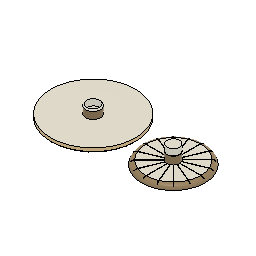
CAKE TABLE (Autodesk Fusion 360 design; units mm, degrees)
part number: 2026-07-16-17-54-16-538
Autodesk Fusion 360 part; units mm, degrees
sketch "Sketch1" plane through (0, 0, 0) normal (0, 1, 0) x (1, 0, 0)
  circle A0 centre (0, 0) radius 75
  dimension "d1" = 150
  constraint coincident A0.centre origin
  measures "d1" diameter of A0
extrude "Extrude1" add sketch "Sketch1" along normal blind 10 makes body 1
ref_plane "WorkPlane1" through (0, 10, 0) normal (0, 1, 0) x (1, 0, 0)
sketch "Sketch2" plane through (0, 10, 0) normal (0, 1, 0) x (1, 0, 0)
  line L0 (0, 0) -> (1, 0)
  line L1 (1, 0) -> (1, -74.9885)
  line L2 (1, -74.9885) -> (0, -74.9885)
  line L3 (0, -74.9885) -> (0, 0)
  line L4 (28.6969, -69.2803) -> (0, 0)
  line L5 (0, 0) -> (0.9239, 0.3827)
  line L6 (29.6207, -68.8977) -> (28.6969, -69.2803)
  line L7 (0.9239, 0.3827) -> (29.6207, -68.8977)
  line L8 (53.0249, -53.0249) -> (0, 0)
  line L9 (0, 0) -> (0.7071, 0.7071)
  line L10 (53.732, -52.3178) -> (53.0249, -53.0249)
  line L11 (0.7071, 0.7071) -> (53.732, -52.3178)
  line L12 (69.2803, -28.6969) -> (0, 0)
  line L13 (0, 0) -> (0.3827, 0.9239)
  line L14 (69.663, -27.773) -> (69.2803, -28.6969)
  line L15 (0.3827, 0.9239) -> (69.663, -27.773)
  line L16 (74.9885, 0) -> (0, 0)
  line L17 (0, 0) -> (0, 1)
  line L18 (74.9885, 1) -> (74.9885, 0)
  line L19 (0, 1) -> (74.9885, 1)
  line L20 (69.2803, 28.6969) -> (0, 0)
  line L21 (0, 0) -> (-0.3827, 0.9239)
  line L22 (68.8977, 29.6207) -> (69.2803, 28.6969)
  line L23 (-0.3827, 0.9239) -> (68.8977, 29.6207)
  line L24 (53.0249, 53.0249) -> (0, 0)
  line L25 (0, 0) -> (-0.7071, 0.7071)
  line L26 (52.3178, 53.732) -> (53.0249, 53.0249)
  line L27 (-0.7071, 0.7071) -> (52.3178, 53.732)
  line L28 (28.6969, 69.2803) -> (0, 0)
  line L29 (0, 0) -> (-0.9239, 0.3827)
  line L30 (27.773, 69.663) -> (28.6969, 69.2803)
  line L31 (-0.9239, 0.3827) -> (27.773, 69.663)
  line L32 (0, 74.9885) -> (0, 0)
  line L33 (0, 0) -> (-1, 0)
  line L34 (-1, 74.9885) -> (0, 74.9885)
  line L35 (-1, 0) -> (-1, 74.9885)
  line L36 (-28.6969, 69.2803) -> (0, 0)
  line L37 (0, 0) -> (-0.9239, -0.3827)
  line L38 (-29.6207, 68.8977) -> (-28.6969, 69.2803)
  line L39 (-0.9239, -0.3827) -> (-29.6207, 68.8977)
  line L40 (-53.0249, 53.0249) -> (0, 0)
  line L41 (0, 0) -> (-0.7071, -0.7071)
  line L42 (-53.732, 52.3178) -> (-53.0249, 53.0249)
  line L43 (-0.7071, -0.7071) -> (-53.732, 52.3178)
  line L44 (-69.2803, 28.6969) -> (0, 0)
  line L45 (0, 0) -> (-0.3827, -0.9239)
  line L46 (-69.663, 27.773) -> (-69.2803, 28.6969)
  line L47 (-0.3827, -0.9239) -> (-69.663, 27.773)
  line L48 (-74.9885, 0) -> (0, 0)
  line L49 (0, 0) -> (0, -1)
  line L50 (-74.9885, -1) -> (-74.9885, 0)
  line L51 (0, -1) -> (-74.9885, -1)
  line L52 (-69.2803, -28.6969) -> (0, 0)
  line L53 (0, 0) -> (0.3827, -0.9239)
  line L54 (-68.8977, -29.6207) -> (-69.2803, -28.6969)
  line L55 (0.3827, -0.9239) -> (-68.8977, -29.6207)
  line L56 (-53.0249, -53.0249) -> (0, 0)
  line L57 (0, 0) -> (0.7071, -0.7071)
  line L58 (-52.3178, -53.732) -> (-53.0249, -53.0249)
  line L59 (0.7071, -0.7071) -> (-52.3178, -53.732)
  line L60 (-28.6969, -69.2803) -> (0, 0)
  line L61 (0, 0) -> (0.9239, -0.3827)
  line L62 (-27.773, -69.663) -> (-28.6969, -69.2803)
  line L63 (0.9239, -0.3827) -> (-27.773, -69.663)
  dimension "d5" = 1
  dimension "d7" = 360
  constraint horizontal L0
  constraint vertical L1
  constraint horizontal L2
  constraint vertical L3
  constraint coincident L0.start L3.end
  measures "d5" distance of L0.start L0.end
extrude "Extrude2" cut sketch "Sketch2" against normal blind 3 contours L1 L4 L6 L7 L8 | L7 L8 L10 L11 L12 | L11 L12 L14 L15 L16 | L3 L59 L60 L62 L63 | L55 L56 L58 L59 L60 | L51 L52 L54 L55 L56 | L1 L2 L3 L4 L63 | L15 L16 L18 L19 L20 | L19 L20 L22 L23 L24 | L23 L24 L26 L27 L28 | L27 L28 L30 L31 L32 | L31 L32 L34 L35 L36 | L35 L36 L38 L39 L40 | L39 L40 L42 L43 L44 | L43 L44 L46 L47 L48 | L47 L48 L50 L51 L52 bodies 1
sketch "Sketch3" plane through (0, 10, 0) normal (0, 1, 0) x (1, 0, 0)
  circle A0 centre (0, 0) radius 15
  dimension "d10" = 30
  constraint coincident A0.centre origin
  measures "d10" diameter of A0
extrude "Extrude3" add sketch "Sketch3" along normal blind 20 separate body makes body 2
fillet "Fillet1" radius 10.5 1 edges at (-69.9246, 10, 27.1212) on bodies 1
move_body "Move1" bodies 2 to x (1, 0, 0) y (0, 1, 0) z (0, 0, 1) at (0, -5, 0)
ref_plane "WorkPlane2" through (0, 30, 0) normal (0, 1, 0) x (1, 0, 0)
sketch "Sketch4" plane through (0, 30, 0) normal (0, 1, 0) x (1, 0, 0)
  circle A0 centre (0, 0) radius 17.5
  dimension "d18" = 35
  constraint coincident A0.centre origin
  measures "d18" diameter of A0
extrude "Extrude4" add sketch "Sketch4" along normal blind 20 separate body makes body 3
fillet "Fillet3" radius 3.5 1 edges at (-16.3157, 30, 6.3283) on bodies 3
move_body "Move2" bodies 3 to x (1, 0, 0) y (0, 1, 0) z (0, 0, 1) at (0, -2, 0)
extrude "Extrude5" add 1 faces at (3.8315, 25, -5.6199) along direction (0, 1, 0) blind 9 on bodies 2 bodies 2 3
ref_plane "WorkPlane3" through (0, 48, 0) normal (0, 1, 0) x (1, 0, 0)
sketch "Sketch5" plane through (0, 48, 0) normal (0, 1, 0) x (1, 0, 0)
  circle A0 centre (0, 0) radius 99.8908
  constraint coincident A0.centre origin
extrude "Extrude6" add sketch "Sketch5" along normal blind 10 separate body makes body 4
fillet "Fillet4" radius 2.5 1 edges at (-93.1309, 58, 36.1221) on bodies 4
ref_plane "WorkPlane4" through (0, 58, 0) normal (0, 1, 0) x (1, 0, 0)
sketch "Sketch6" plane through (0, 58, 0) normal (0, 1, 0) x (1, 0, 0)
  circle A0 centre (0, 0) radius 17.4885
  circle A1 centre (0, 0) radius 16.8218
  line L0 (0.5452, -17.48) -> (-1.5075, -17.48)
  line L1 (-1.5075, -17.48) -> (-1.5075, -98.7314)
  line L2 (-1.5075, -98.7314) -> (0.5452, -98.7314)
  line L3 (0.5452, -98.7314) -> (0.5452, -17.48)
  line L4 (63.881, -75.2822) -> (11.6536, -13.04)
  line L5 (11.6536, -13.04) -> (10.0812, -14.3595)
  line L6 (10.0812, -14.3595) -> (62.3085, -76.6017)
  line L7 (62.3085, -76.6017) -> (63.881, -75.2822)
  line L8 (97.3262, -16.6076) -> (17.3092, -2.4985)
  line L9 (17.3092, -2.4985) -> (16.9527, -4.52)
  line L10 (16.9527, -4.52) -> (96.9697, -18.6291)
  line L11 (96.9697, -18.6291) -> (97.3262, -16.6076)
  line L12 (85.2313, 49.8379) -> (14.8656, 9.2122)
  line L13 (14.8656, 9.2122) -> (15.8919, 7.4345)
  line L14 (15.8919, 7.4345) -> (86.2577, 48.0602)
  line L15 (86.2577, 48.0602) -> (85.2313, 49.8379)
  line L16 (33.2558, 92.9637) -> (5.4662, 16.6123)
  line L17 (5.4662, 16.6123) -> (7.3951, 15.9103)
  line L18 (7.3951, 15.9103) -> (35.1847, 92.2616)
  line L19 (35.1847, 92.2616) -> (33.2558, 92.9637)
  line L20 (-34.2805, 92.5907) -> (-6.4909, 16.2394)
  line L21 (-6.4909, 16.2394) -> (-4.562, 16.9415)
  line L22 (-4.562, 16.9415) -> (-32.3516, 93.2928)
  line L23 (-32.3516, 93.2928) -> (-34.2805, 92.5907)
  line L24 (-85.7765, 48.8935) -> (-15.4108, 8.2679)
  line L25 (-15.4108, 8.2679) -> (-14.3844, 10.0455)
  line L26 (-14.3844, 10.0455) -> (-84.7502, 50.6712)
  line L27 (-84.7502, 50.6712) -> (-85.7765, 48.8935)
  line L28 (-97.1368, -17.6815) -> (-17.1198, -3.5723)
  line L29 (-17.1198, -3.5723) -> (-17.4763, -1.5508)
  line L30 (-17.4763, -1.5508) -> (-97.4932, -15.6599)
  line L31 (-97.4932, -15.6599) -> (-97.1368, -17.6815)
  line L32 (-63.0457, -75.9831) -> (-10.8183, -13.7409)
  line L33 (-10.8183, -13.7409) -> (-12.3908, -12.4215)
  line L34 (-12.3908, -12.4215) -> (-64.6181, -74.6637)
  line L35 (-64.6181, -74.6637) -> (-63.0457, -75.9831)
  dimension "d33" = 360
  constraint coincident A0.centre A1.centre
  constraint concentric A0 A1
  constraint horizontal L0
  constraint vertical L1
  constraint horizontal L2
  constraint vertical L3
  constraint coincident A0 L0.start
extrude "Extrude7" cut sketch "Sketch6" against normal blind 1 contours A0 L8 L9 L10 L11 | A0 L12 L13 L14 L15 | A0 L4 L5 L6 L7 | A0 L16 L17 L18 L19 | A0 L0 L1 L2 L3 | A0 L20 L21 L22 L23 | A0 L32 L33 L34 L35 | A0 L24 L25 L26 L27 | A0 L28 L29 L30 L31 bodies 4
extrude "Extrude8" cut sketch "Sketch6" against normal blind 0.5 contours A0 L0 L5 L9 L13 L17 L21 L25 L29 L33 bodies 4
sketch "Sketch7" plane through (0, 58, 0) normal (0, 1, 0) x (1, 0, 0)
  circle A0 centre (0, 37.1794) radius 4.1177
  circle A1 centre (-23.8985, 28.4811) radius 4.1177
  circle A2 centre (-36.6146, 6.4561) radius 4.1177
  circle A3 centre (-32.1983, -18.5897) radius 4.1177
  circle A4 centre (-12.7161, -34.9372) radius 4.1177
  circle A5 centre (12.7161, -34.9372) radius 4.1177
  circle A6 centre (32.1983, -18.5897) radius 4.1177
  circle A7 centre (36.6146, 6.4561) radius 4.1177
  circle A8 centre (23.8985, 28.4811) radius 4.1177
  line L0 (-10.6484, 80) -> (-10.6484, 84.3604)
  line L1 (10, 84.3604) -> (10, 80)
  arc A9 (10, 80) -> (-10.6484, 80) centre (-0.3242, 59.8184) ccw
  arc A10 (10, 84.3604) -> (-10.6484, 84.3604) centre (-0.3242, 70.6427) ccw
  arc A11 (-46.5654, 71.0517) -> (-62.383, 57.7791) centre (-45.6566, 53.9071) ccw
  line L2 (-46.5654, 71.0517) -> (-43.7626, 67.7114)
  arc A12 (-43.7626, 67.7114) -> (-59.5802, 54.4389) centre (-38.6989, 45.6151) ccw
  line L3 (-59.5802, 54.4389) -> (-62.383, 57.7791)
  arc A13 (-81.3423, 24.4971) -> (-84.9278, 4.1624) centre (-69.6258, 11.9477) ccw
  line L4 (-81.3423, 24.4971) -> (-77.0481, 23.7399)
  arc A14 (-77.0481, 23.7399) -> (-80.6337, 3.4052) centre (-58.9659, 10.0681) ccw
  line L5 (-80.6337, 3.4052) -> (-84.9278, 4.1624)
  arc A15 (-78.0582, -33.5199) -> (-67.734, -51.402) centre (-61.0163, -35.6022) ccw
  line L6 (-78.0582, -33.5199) -> (-74.282, -31.3397)
  arc A16 (-74.282, -31.3397) -> (-63.9578, -49.2218) centre (-51.6421, -30.19) ccw
  line L7 (-63.9578, -49.2218) -> (-67.734, -51.402)
  arc A17 (-38.2499, -75.8526) -> (-18.8467, -82.9148) centre (-23.8566, -66.4934) ccw
  line L8 (-38.2499, -75.8526) -> (-36.7585, -71.7552)
  arc A18 (-36.7585, -71.7552) -> (-17.3554, -78.8174) centre (-20.1544, -56.3218) ccw
  line L9 (-17.3554, -78.8174) -> (-18.8467, -82.9148)
  arc A19 (19.456, -82.693) -> (38.8592, -75.6308) centre (24.4659, -66.2716) ccw
  line L10 (19.456, -82.693) -> (17.9647, -78.5956)
  arc A20 (17.9647, -78.5956) -> (37.3679, -71.5334) centre (20.7638, -56.1) ccw
  line L11 (37.3679, -71.5334) -> (38.8592, -75.6308)
  arc A21 (68.0582, -50.8404) -> (78.3824, -32.9584) centre (61.3405, -35.0406) ccw
  line L12 (68.0582, -50.8404) -> (64.282, -48.6603)
  arc A22 (64.282, -48.6603) -> (74.6063, -30.7782) centre (51.9663, -29.6284) ccw
  line L13 (74.6063, -30.7782) -> (78.3824, -32.9584)
  arc A23 (84.8152, 4.8009) -> (81.2297, 25.1357) centre (69.5132, 12.5863) ccw
  line L14 (84.8152, 4.8009) -> (80.5211, 4.0438)
  arc A24 (80.5211, 4.0438) -> (76.9355, 24.3785) centre (58.8533, 10.7066) ccw
  line L15 (76.9355, 24.3785) -> (81.2297, 25.1357)
  arc A25 (61.8862, 58.1959) -> (46.0686, 71.4685) centre (45.1599, 54.3239) ccw
  line L16 (61.8862, 58.1959) -> (59.0835, 54.8557)
  arc A26 (59.0835, 54.8557) -> (43.2658, 68.1282) centre (38.2021, 46.0319) ccw
  line L17 (43.2658, 68.1282) -> (46.0686, 71.4685)
  dimension "d39" = 360
  dimension "d41" = 360
  constraint vertical L0
  constraint vertical L1
extrude "Extrude9" cut sketch "Sketch7" against normal blind 1 bodies 4
combine "Combine1" operation add target body 1 tool bodies 2 4
ref_plane "WorkPlane5" through (0, 28, 0) normal (0, 1, 0) x (0, 0, 1)
split "Split1" by plane through (0, 28, 0) normal (0, 1, 0) bodies 1 makes body 5 at (71.9902, 48, 5.8321)
move_body "Move3" bodies 5 to x (-1, 0, 0) y (0, -1, 0) z (0, 0, 1) at (-199.7816, 56, 0)
move_body "Align1" bodies 5 to x (1, 0, 0) y (0, 1, 0) z (0, 0, 1) at (199.7816, 2, 0)
move_body "Move4" bodies 5 to x (1, 0, 0) y (0, 1, 0) z (0, 0, 1) at (-190, 0, 0)
extrude "Extrude10" cut 1 faces at (-180.7173, 30, 3.6432) along direction (0, -1, 0) blind 15 on bodies 5 bodies 5
sketch "Sketch8" plane through (0, 28, 0) normal (0, 1, 0) x (-1, 0, 0)
  circle A0 centre (0, 0) radius 15
  circle A1 centre (0, 0) radius 14.5
  dimension "d47" = 29
  constraint concentric A0 A1
  measures "d47" diameter of A1
extrude "Extrude11" add sketch "Sketch8" along normal blind 15 contours A1 bodies 1
named bodies: "BASE", "TOP"
